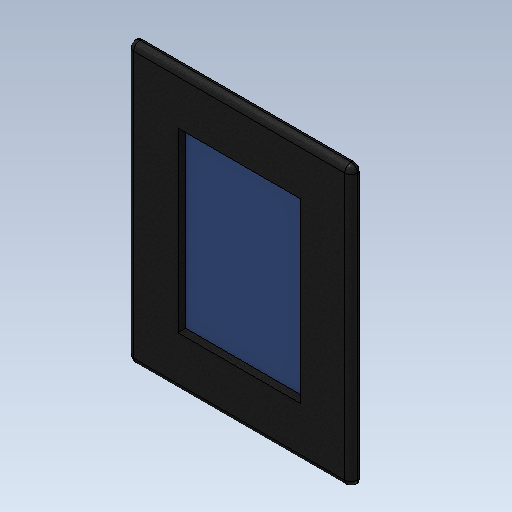
# Autodesk Inventor part: Control Panel
Saved by Autodesk Inventor 2020.1 (Build 241239000, 239)
## iProperties
Created: 2009-10-16
Part Number: Control Panel
Document SubType Name: Modeling
Designer: Thom Tremblay
Density: 1 g/cm^3
Material: Generic
Appearance: Black Cast
Author: Thom Tremblay
Autodesk Inventor part; units mm, degrees
ref_plane "YZ Plane" through (0, 0, 0) normal (1, 0, 0) x (0, 1, 0)
ref_plane "XZ Plane" through (0, 0, 0) normal (0, 1, 0) x (-1, 0, 0)
ref_plane "XY Plane" through (0, 0, 0) normal (0, 0, 1) x (1, 0, 0)
sketch "Sketch1" plane through (0, 0, 0) normal (0, 0, 1) x (1, 0, 0)
  line L0 (111.0996, -138.3538) -> (-111.0996, -138.3538)
  line L1 (-111.0996, -138.3538) -> (-111.0996, 138.3538)
  line L2 (-111.0996, 138.3538) -> (111.0996, 138.3538)
  line L3 (111.0996, 138.3538) -> (111.0996, -138.3538)
  point P0 (0, 0)
  point P1 (111.0996, 0)
  point P2 (0, -138.3538)
  dimension "d0" = 276.7076
  dimension "d1" = 222.1992
  constraints: 8 end point, 2 midpoint, 2 parallel, 1 horizontal, 1 horizontal alignment, 1 perpendicular, 1 vertical alignment
  measures "d0" distance of L2.end L0.start
  measures "d1" distance of L0.start L0.end
extrude "Extrusion1" add sketch "Sketch1" along normal blind 8.001
sketch "Sketch2" plane through (0, 0, 8.001) normal (0, 0, 1) x (1, 0, 0)
  line L0 (-111.0996, -138.3538) -> (-111.0996, 138.3538) construction
  line L1 (111.0996, -138.3538) -> (-111.0996, -138.3538) construction
  line L2 (111.0996, 138.3538) -> (111.0996, -138.3538) construction
  line L3 (-111.0996, 138.3538) -> (111.0996, 138.3538) construction
  line L4 (56.9107, -84.1649) -> (-56.9107, -84.1649)
  line L5 (-56.9107, -84.1649) -> (-56.9107, 84.1649)
  line L6 (-56.9107, 84.1649) -> (56.9107, 84.1649)
  line L7 (56.9107, 84.1649) -> (56.9107, -84.1649)
  point P0 (0, 0)
  dimension "d4" = 203.2
  constraints: 8 end point, 3 other
  measures "d4" distance of L4.start L5.end
extrude "Extrusion2" cut sketch "Sketch2" against normal blind 3.81
draft "FaceDraft1" angle 45 pull direction (0, 0, 1) faces at (56.9107, 28.055, 6.731) (18.9702, -84.1649, 6.731) (-56.9107, -28.055, 6.731) (-18.9702, 84.1649, 6.731) fixed edges at (56.9107, 0, 4.191) (0, -84.1649, 4.191) (-56.9107, 0, 4.191) (0, 84.1649, 4.191)
fillet "Fillet1" radius 6.35 8 edges at (-111.0996, 0, 8.001) (0, -138.3538, 8.001) (111.0996, 0, 8.001) (0, 138.3538, 8.001) (-111.0996, 138.3538, 4.0005) (111.0996, 138.3538, 4.0005) (111.0996, -138.3538, 4.0005) (-111.0996, -138.3538, 4.0005)
sketch "Sketch3" plane through (0, 0, 0) normal (0, 0, -1) x (-1, 0, 0)
  line L0 (-84.586, 111.4782) -> (84.586, 111.4782)
  line L1 (84.586, 111.4782) -> (84.586, -111.4782)
  line L2 (84.586, -111.4782) -> (-84.586, -111.4782)
  line L3 (-84.586, -111.4782) -> (-84.586, 111.4782)
  point P0 (0, 0)
  point P1 (84.586, 0)
  point P2 (0, -111.4782)
  constraints: 8 end point, 2 midpoint, 2 parallel, 1 horizontal, 1 horizontal alignment, 1 perpendicular, 1 vertical alignment
extrude "Extrusion3" add sketch "Sketch3" along normal blind 25.4
sketch "Sketch4" plane through (-84.586, -111.4782, 0) normal (-1, 0, 0) x (0, 0, 1)
  line L0 (-17.78, 159.4565) -> (-11.43, 159.4565)
  line L1 (-11.43, 159.4565) -> (-11.43, 141.6765)
  line L2 (-11.43, 141.6765) -> (-17.78, 141.6765)
  line L3 (-17.78, 141.6765) -> (-17.78, 159.4565)
  point P0 (0, 111.4782)
  point P1 (-25.4, 222.9565)
  dimension "d11" = 17.78
  dimension "d12" = 6.35
  dimension "d33" = 63.5
  dimension "d34" = 7.62
  constraints: 8 end point, 2 parallel, 1 horizontal, 1 perpendicular
  measures "d11" distance of L2.end L0.start
  measures "d12" distance of L0.start L0.end
  measures "d33" distance from line of point (-25.4, 222.956) L0
  measures "d34" distance from line of point (-25.4, 222.956) L3
extrude "Extrusion4" cut sketch "Sketch4" against normal blind 6.35
sketch "Sketch5" plane through (-78.236, -111.4782, 0) normal (-1, 0, 0) x (0, 0, 1)
  line L0 (-13.0302, 145.5881) -> (-13.0302, 144.9531)
  line L1 (-13.0302, 144.9531) -> (-13.6652, 144.9531)
  line L2 (-13.6652, 144.9531) -> (-13.6652, 145.5881)
  line L3 (-13.6652, 145.5881) -> (-13.0302, 145.5881)
  line L4 (-11.43, 141.6765) -> (-11.43, 159.4565) projected
  line L5 (-17.78, 141.6765) -> (-11.43, 141.6765) projected
  point P0 (0, 111.4782)
  point P1 (-13.3477, 145.2706)
  dimension "d15" = 0.635
  dimension "d16" = 1.6002
  dimension "d17" = 3.2766
  constraints: 8 end point, 1 vertical, 9 other
  measures "d15" distance of L0.start L0.end
  measures "d16" distance between parallel lines of L4 L0
  measures "d17" distance from line of L1.end L5
extrude "Extrusion5" add sketch "Sketch5" along normal blind 6.096
chamfer "Chamfer1" distance 0.1524 angle 45 4 edges at (-84.332, 33.7923, -13.0302) (-84.332, 33.4748, -13.3477) (-84.332, 33.7923, -13.6652) (-84.332, 34.1098, -13.3477)
pattern_linear "Rectangular Pattern1" count 5 spacing 2.6416 along (0, 1, 0) count 2 spacing 2.6416 along (0, 0, -1) of "Extrusion5", "Chamfer1"
sketch "Sketch6" plane through (-84.586, -111.4782, 0) normal (-1, 0, 0) x (0, 0, 1)
  line L0 (-10.16, 153.6653) -> (-11.43, 153.6653)
  line L1 (-11.43, 153.6653) -> (-11.43, 147.4677)
  line L2 (-11.43, 147.4677) -> (-10.16, 147.4677)
  line L3 (-10.16, 147.4677) -> (-10.16, 153.6653)
  line L4 (-11.43, 159.4565) -> (-11.43, 141.6765) projected
  point P0 (0, 111.4782)
  point P1 (-11.43, 150.5665)
  dimension "d29" = 6.1976
  dimension "d30" = 1.27
  constraints: 8 end point, 2 midpoint, 2 parallel, 1 horizontal, 1 perpendicular
  measures "d29" distance of L2.end L0.start
  measures "d30" distance of L1.end L2.end
extrude "Extrusion6" cut sketch "Sketch6" against normal up to surface (6.35 mm away)
body "Solid1"
